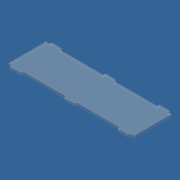
# Autodesk Inventor part: P1704_102
Saved by Autodesk Inventor 2015 (Build 190159000, 159)
## iProperties
Created: 2017-02-08
Part Number: P1704_102
Project: Manette
Material: Plastique PMMA
Description: Paroi arrière - Chevalier
Document SubType Name: Modeling
Designer: Alexandre.PICOTTE
Authority: 172x58x3
Density: 1.188 g/cm^3
Appearance: Transparent - Clair
Mass: 33.5334 g
Surface Area: 203.216 cm^2
Volume: 28.2268 cm^3
Material number: ---
Author: Boris.GAUDARD
Autodesk Inventor part; units mm, degrees
ref_plane "Plan YZ" through (0, 0, 0) normal (1, 0, 0) x (0, 1, 0)
ref_plane "Plan XZ" through (0, 0, 0) normal (0, 1, 0) x (-1, 0, 0)
ref_plane "Plan XY" through (0, 0, 0) normal (0, 0, 1) x (1, 0, 0)
sketch "Esquisse7" plane through (0, 0, 0) normal (0, 0, 1) x (1, 0, 0)
  line L0 (-88, -26) -> (-88, 26)
  line L1 (-88, 26) -> (-83, 26)
  line L2 (-83, 26) -> (-83, 29)
  line L3 (-83, 29) -> (-68, 29)
  line L4 (-68, 29) -> (-68, 26)
  line L5 (-68, 26) -> (-7.5, 26)
  line L6 (-7.5, 26) -> (-7.5, 29)
  line L7 (-7.5, 29) -> (7.5, 29)
  line L8 (7.5, 29) -> (7.5, 26)
  line L9 (7.5, 26) -> (68, 26)
  line L10 (68, 26) -> (68, 29)
  line L11 (68, 29) -> (83, 29)
  line L12 (83, 29) -> (83, 26)
  line L13 (83, 26) -> (88, 26)
  line L14 (88, 26) -> (88, -26)
  line L15 (88, -26) -> (83, -26)
  line L16 (83, -26) -> (83, -29)
  line L17 (83, -29) -> (68, -29)
  line L18 (68, -29) -> (68, -26)
  line L19 (7.5, -26) -> (7.5, -29)
  line L20 (7.5, -26) -> (68, -26)
  line L21 (7.5, -29) -> (-7.5, -29)
  line L22 (-7.5, -29) -> (-7.5, -26)
  line L23 (-7.5, -26) -> (-68, -26)
  line L24 (-68, -26) -> (-68, -29)
  line L25 (-68, -29) -> (-83, -29)
  line L26 (-83, -29) -> (-83, -26)
  line L27 (-83, -26) -> (-88, -26)
  line L28 (0, -40.6) -> (0, 40.6) construction
  line L29 (-123.2, 0) -> (123.2, 0) construction
  dimension "d33" = 52
  dimension "d34" = 15
  dimension "d35" = 3
  dimension "d36" = 5
  dimension "d65" = 176
  constraints: 56 end point, 24 point on line, 15 perpendicular, 7 equal length, 2 horizontal, 1 vertical, 3 other
  measures "d33" distance of L0.start L0.end
  measures "d34" distance of L2.end L3.end
  measures "d35" distance of L1.end L2.end
  measures "d36" distance of L0.end L1.end
  measures "d65" distance between parallel lines of L14 L0
extrude "Extrusion2" add sketch "Esquisse7" against normal blind 3
sketch "Esquisse8" plane through (0, 0, 0) normal (0, 0, 1) x (1, 0, 0)
  point P0 (0, 0)
  point P1 (7.5, 26)
  point P2 (-7.5, 26)
  point P3 (-83, 26)
  point P4 (-68, 26)
  point P5 (-83, -26)
  point P6 (-68, -26)
  point P7 (-7.5, -26)
  point P8 (7.5, -26)
  point P9 (68, -26)
  point P10 (83, -26)
  point P11 (68, 26)
  point P12 (83, 26)
  point P13 (83, 26)
  point P14 (68, -26)
  point P15 (83, 26)
  constraints: 3 coincident
hole "Perçage2" at (7.5, 26, 0) at (-7.5, 26, 0) at (-83, 26, 0) at (-68, 26, 0) at (-83, -26, 0) at (-68, -26, 0) at (-7.5, -26, 0) at (7.5, -26, 0) at (68, -26, 0) at (83, -26, 0) at (68, 26, 0) at (83, 26, 0) direction (0, 0, -1) diameter 1 end through all
chamfer "Chanfrein3" distance 1 angle 45 12 edges at (-83, -29, -1.5) (-68, -29, -1.5) (-83, 29, -1.5) (-68, 29, -1.5) (-7.5, 29, -1.5) (7.5, 29, -1.5) (68, 29, -1.5) (83, 29, -1.5) (68, -29, -1.5) (83, -29, -1.5) (-7.5, -29, -1.5) (7.5, -29, -1.5)
